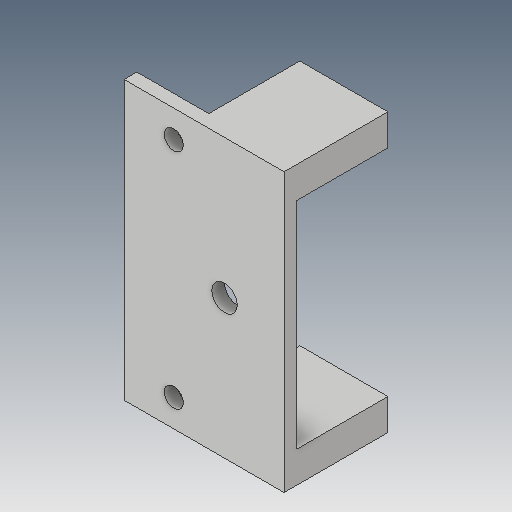
# Autodesk Inventor part: 20_focus_inlet_plate_bottom
Saved by Autodesk Inventor 2019.4 (Build 234330000, 330)
## iProperties
Created: 2020-02-05
Part Number: 20_focus_inlet_plate_bottom
Material: Generic
Document SubType Name: Modeling
Designer: marsikovabarbora
Density: 1 g/cm^3
Appearance: Default
Author: marsikovabarbora
Autodesk Inventor part; units mm, degrees
ref_plane "YZ Plane" through (0, 0, 0) normal (1, 0, 0) x (0, 1, 0)
sketch "Sketch1" plane through (0, 0, 0) normal (0, 0, 1) x (1, 0, 0)
  line L0 (8.6463, -3.6882) -> (-2.6463, -3.6882) construction
  line L1 (8.6463, 3.6882) -> (8.6463, -3.6882) construction
  line L2 (-2.6463, 3.6882) -> (8.6463, 3.6882) construction
  circle A0 centre (5.1537, -0.6118) radius 1.4 construction
  line L3 (-2.6463, -39.9118) -> (8.6463, -39.9118) construction
  line L4 (8.6463, -39.9118) -> (8.6463, -32.5353) construction
  line L5 (8.6463, -32.5353) -> (-2.6463, -32.5353) construction
  circle A1 centre (5.1537, -35.6118) radius 1.4 construction
  line L6 (8.6463, -35.0118) -> (8.6463, -39.9118) construction
  line L7 (8.6463, -39.9118) -> (25.0537, -39.9118) construction
  line L8 (74.7537, -39.9118) -> (74.7537, -34.8118) construction
  line L9 (74.7537, -34.8118) -> (70.7537, -34.8118) construction
  line L10 (70.7537, -34.8118) -> (70.7537, -35.0118) construction
  line L11 (23.2537, -35.0118) -> (8.6463, -35.0118) construction
  line L12 (8.6463, 3.6882) -> (8.6463, -1.2118) construction
  line L13 (8.6463, -1.2118) -> (23.2537, -1.2118) construction
  line L14 (70.7537, -1.2118) -> (70.7537, -1.4118) construction
  line L15 (70.7537, -1.4118) -> (74.7537, -1.4118) construction
  line L16 (74.7537, -1.4118) -> (74.7537, 3.6882) construction
  line L17 (25.0537, 3.6882) -> (8.6463, 3.6882) construction
  line L18 (19.9537, -11.1118) -> (9.9537, -11.1118) construction
  line L19 (9.9537, -16.4118) -> (9.9537, -11.1118) construction
  line L20 (19.9537, -16.4118) -> (9.9537, -16.4118) construction
  line L21 (19.9537, -16.4118) -> (19.9537, -11.1118) construction
  line L22 (-2.6463, 3.6882) -> (22.4609, 3.6882)
  line L23 (22.4609, 3.6882) -> (22.4609, -39.9118)
  line L24 (22.4609, -39.9118) -> (-2.6463, -39.9118)
  line L25 (-2.6463, -39.9118) -> (-2.6463, 3.6882)
  circle A2 centre (5.1537, -0.6118) radius 1.5
  circle A3 centre (5.1537, -35.6118) radius 1.5
  line L26 (14.5908, -13.5618) -> (14.5908, -11.1118) construction
  line L27 (11.6908, -13.5618) -> (11.6908, -11.1118) construction
  line L28 (14.5908, -25.1118) -> (14.5908, -22.6618) construction
  line L29 (11.6908, -25.1118) -> (11.6908, -22.6618) construction
  circle A4 centre (13.1145, -18.1118) radius 2
  line L30 (-2.6463, -32.5353) -> (-2.6463, -39.9118) projected
  line L31 (34.9537, -32.1118) -> (26.1537, -32.1118) projected
  line L32 (23.2537, -35.0118) -> (26.1537, -32.1118) projected
  line L33 (25.0537, -39.9118) -> (25.0537, -39.3319) projected
  line L34 (26.7161, -37.6695) -> (25.0537, -39.3319) projected
  arc A5 (27.8115, -36.5741) -> (26.7161, -37.6695) centre (28.2537, -38.1118) ccw projected
  line L35 (29.4557, -34.9299) -> (27.8115, -36.5741) projected
  line L36 (36.8518, -34.9299) -> (29.4557, -34.9299) projected
  line L37 (38.496, -36.5741) -> (36.8518, -34.9299) projected
  arc A6 (39.5914, -37.6695) -> (38.496, -36.5741) centre (38.0537, -38.1118) ccw projected
  line L38 (41.2537, -39.3319) -> (39.5914, -37.6695) projected
  line L39 (41.2537, -39.3319) -> (41.2537, -39.9118) projected
  line L40 (41.2537, -39.9118) -> (74.7537, -39.9118) projected
  line L41 (70.7537, -35.0118) -> (44.2537, -35.0118) projected
  line L42 (41.2537, -32.0118) -> (44.2537, -35.0118) projected
  line L43 (34.9537, -32.0118) -> (41.2537, -32.0118) projected
  line L44 (34.9537, -32.0118) -> (34.9537, -32.1118) projected
  line L45 (34.9537, -4.1118) -> (34.9537, -4.2118) projected
  line L46 (34.9537, -4.2118) -> (41.2537, -4.2118) projected
  line L47 (41.2537, -4.2118) -> (44.2537, -1.2118) projected
  line L48 (44.2537, -1.2118) -> (70.7537, -1.2118) projected
  line L49 (74.7537, 3.6882) -> (41.2537, 3.6882) projected
  line L50 (41.2537, 3.6882) -> (41.2537, 3.1083) projected
  line L51 (41.2537, 3.1083) -> (39.5914, 1.446) projected
  arc A7 (38.496, 0.3506) -> (39.5914, 1.446) centre (38.0537, 1.8882) ccw projected
  line L52 (38.496, 0.3506) -> (36.8518, -1.2936) projected
  line L53 (36.8518, -1.2936) -> (29.4557, -1.2936) projected
  line L54 (29.4557, -1.2936) -> (27.8115, 0.3506) projected
  arc A8 (26.7161, 1.446) -> (27.8115, 0.3506) centre (28.2537, 1.8882) ccw projected
  line L55 (26.7161, 1.446) -> (25.0537, 3.1083) projected
  line L56 (25.0537, 3.1083) -> (25.0537, 3.6882) projected
  line L57 (23.2537, -1.2118) -> (26.1537, -4.1118) projected
  line L58 (26.1537, -4.1118) -> (34.9537, -4.1118) projected
  line L59 (-2.6463, 3.6882) -> (-2.6463, -3.6882) projected
  point P0 (0, 0)
  dimension "d0" = 0.1
  dimension "d1" = 0.1
  dimension "d2" = 4
  constraints: 16 end point, 4 vertical, 3 centre point, 2 parallel, 1 horizontal, 1 perpendicular, 1 point on line, 8 other
  measures "d0" radial gap between concentric circles of A0 A2
  measures "d1" radial gap between concentric circles of A1 A3
  measures "d2" diameter of A4
extrude "Extrusion1" add sketch "Sketch1" along normal blind 2
sketch "Sketch2" plane through (0, 0, 0) normal (0, 0, -1) x (-1, 0, 0)
  circle A0 centre (-13.1145, -18.1118) radius 2 construction
  circle A1 centre (-5.1537, -35.6118) radius 1.5 construction
  circle A2 centre (-5.1537, -0.6118) radius 1.5 construction
  line L0 (2.6463, 3.6882) -> (-22.4609, 3.6882) construction
  line L1 (-22.4609, 3.6882) -> (-22.4609, -39.9118) construction
  line L2 (-22.4609, -39.9118) -> (2.6463, -39.9118) construction
  line L3 (2.6463, -39.9118) -> (2.6463, 3.6882) construction
  line L4 (-8.6463, 3.6882) -> (-8.6463, -3.6882) construction
  line L5 (-8.6463, -39.9118) -> (-8.6463, -32.5353) construction
  line L6 (-8.6463, -1.2118) -> (-23.2537, -1.2118) construction
  line L7 (-8.6463, -35.0118) -> (-23.2537, -35.0118) construction
  line L8 (-22.4609, -39.9118) -> (-8.6463, -39.9118)
  line L9 (-8.6463, -39.9118) -> (-8.6463, -35.0118)
  line L10 (-8.6463, -35.0118) -> (-22.4609, -35.0118)
  line L11 (-22.4609, -35.0118) -> (-22.4609, -39.9118)
  line L12 (-22.4609, -39.9118) -> (-22.4609, 3.6882) projected
  line L13 (-22.4609, -1.2118) -> (-8.6463, -1.2118)
  line L14 (-8.6463, -1.2118) -> (-8.6463, 3.6882)
  line L15 (-8.6463, 3.6882) -> (-22.4609, 3.6882)
  line L16 (-22.4609, 3.6882) -> (-22.4609, -1.2118)
  point P0 (0, 0)
  constraints: 16 end point, 4 parallel, 2 horizontal, 2 perpendicular, 2 point on line
ref_plane "Work Plane1" through (8.6463, -1.4118, -16.3) normal (0, 0, 1) x (1, 0, 0)
ref_plane "Work Plane2" through (8.6463, -39.9118, -14.3) normal (0, 0, 1) x (1, 0, 0)
extrude "Extrusion2" add sketch "Sketch2" along normal up to surface (14.3 mm away)
body "Solid1"
